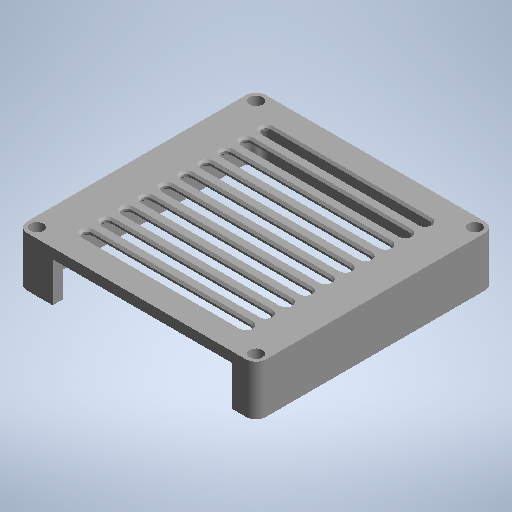
# Autodesk Inventor part: Part6
Saved by Autodesk Inventor 2025.4 (Build 294407000, 407)
## iProperties
Created: 2026-08-04
Part Number: Part6
Material: Générique
Document SubType Name: Modeling
Designer: louis
Density: 1 g/cm^3
Appearance: Par défaut
Author: louis
Autodesk Inventor part; units mm, degrees
ref_plane "YZ Plane" through (0, 0, 0) normal (1, 0, 0) x (0, 1, 0)
ref_plane "XZ Plane" through (0, 0, 0) normal (0, 1, 0) x (-1, 0, 0)
ref_plane "XY Plane" through (0, 0, 0) normal (0, 0, 1) x (1, 0, 0)
sketch "Sketch2" plane through (0, 0, 0) normal (0, 0, 1) x (1, 0, 0)
  line L0 (-55, -60) -> (55, -60)
  line L1 (60, -55) -> (60, 55)
  line L2 (55, 60) -> (-55, 60)
  line L3 (-60, 55) -> (-60, -55)
  line L4 (-60, -60) -> (60, 60) construction
  line L5 (60, -60) -> (-60, 60) construction
  arc A0 (-55, 60) -> (-60, 55) centre (-55, 55) ccw
  arc A1 (60, 55) -> (55, 60) centre (55, 55) ccw
  arc A2 (55, -60) -> (60, -55) centre (55, -55) ccw
  arc A3 (-60, -55) -> (-55, -60) centre (-55, -55) ccw
  line L6 (-55, 55) -> (55, 55)
  line L7 (55, 55) -> (55, -55)
  line L8 (55, -55) -> (-55, -55)
  line L9 (-55, -55) -> (-55, 55)
  circle A4 centre (-55, 55) radius 4
  circle A5 centre (55, 55) radius 4
  circle A6 centre (55, -55) radius 4
  circle A7 centre (-55, -55) radius 4
  point P0 (0, 0)
  point P1 (-55, -51)
  point P2 (-55, 51)
  point P3 (-51, 55)
  point P4 (51, 55)
  point P5 (55, 51)
  point P6 (55, -51)
  point P7 (51, -55)
  point P8 (-51, -55)
  dimension "d0" = 120
  dimension "d1" = 120
  dimension "d2" = 5
  dimension "d3" = 5
  dimension "d4" = 5
  dimension "d5" = 8
  dimension "d6" = 8
  dimension "d7" = 8
  dimension "d8" = 8
  constraints: 20 end point, 8 centre point, 8 point on circle, 8 point on line, 8 tangent, 4 coincident, 4 parallel, 2 equal radius, 2 midpoint, 2 perpendicular, 1 horizontal, 3 other
  measures "d0" distance of L5.end L4.end
  measures "d1" distance of L4.end L5.start
  measures "d2" radius of A0
  measures "d3" radius of A1
  measures "d4" distance between parallel lines of L2 L6
  measures "d5" diameter of A4
  measures "d6" diameter of A5
  measures "d7" diameter of A6
  measures "d8" diameter of A7
extrude "Extrusion1" add sketch "Sketch2" along normal blind 22 contours A3 L3 A0 L2 A1 L1 A2 L0 | L9 A4 L6 | L6 A4 L9 | A5 L7 L6 | L6 L7 A5 | A7 L8 L9 | L9 L8 A7 | A6 L8 L7 | L7 L8 A6
fillet "Fillet1" radius 4 8 edges at (-55, -51, 11) (-51, 55, 11) (-55, 51, 11) (-51, -55, 11) (51, -55, 11) (55, -51, 11) (55, 51, 11) (51, 55, 11)
sketch "Sketch4" plane through (0, 0, 22) normal (0, 0, 1) x (1, 0, 0)
  arc A0 (55, -60) -> (60, -55) centre (55, -55) ccw projected
  line L0 (60, -55) -> (60, 55) projected
  arc A1 (60, 55) -> (55, 60) centre (55, 55) ccw projected
  line L1 (55, 60) -> (-55, 60) projected
  arc A2 (-55, 60) -> (-60, 55) centre (-55, 55) ccw projected
  line L2 (-60, 55) -> (-60, -55) projected
  arc A3 (-60, -55) -> (-55, -60) centre (-55, -55) ccw projected
  line L3 (-55, -60) -> (55, -60) projected
  line L4 (-55, -48.0718) -> (-55, 48.0718) projected
  arc A4 (-53, 51.5359) -> (-55, 48.0718) centre (-51, 48.0718) ccw projected
  arc A5 (-53, 51.5359) -> (-51.5359, 53) centre (-55, 55) ccw projected
  arc A6 (-48.0718, 55) -> (-51.5359, 53) centre (-48.0718, 51) ccw projected
  line L5 (-48.0718, 55) -> (48.0718, 55) projected
  arc A7 (51.5359, 53) -> (48.0718, 55) centre (48.0718, 51) ccw projected
  arc A8 (51.5359, 53) -> (53, 51.5359) centre (55, 55) ccw projected
  arc A9 (55, 48.0718) -> (53, 51.5359) centre (51, 48.0718) ccw projected
  line L6 (55, 48.0718) -> (55, -48.0718) projected
  arc A10 (53, -51.5359) -> (55, -48.0718) centre (51, -48.0718) ccw projected
  arc A11 (53, -51.5359) -> (51.5359, -53) centre (55, -55) ccw projected
  arc A12 (48.0718, -55) -> (51.5359, -53) centre (48.0718, -51) ccw projected
  line L7 (48.0718, -55) -> (-48.0718, -55) projected
  arc A13 (-51.5359, -53) -> (-48.0718, -55) centre (-48.0718, -51) ccw projected
  arc A14 (-51.5359, -53) -> (-53, -51.5359) centre (-55, -55) ccw projected
  arc A15 (-55, -48.0718) -> (-53, -51.5359) centre (-51, -48.0718) ccw projected
  line L8 (-40, 45) -> (40, 45) construction
  line L9 (-40, 42.75) -> (40, 42.75)
  line L10 (40, 47.25) -> (-40, 47.25)
  arc A16 (-40, 47.25) -> (-40, 42.75) centre (-40, 45) ccw
  arc A17 (40, 42.75) -> (40, 47.25) centre (40, 45) ccw
  line L11 (0, 0) -> (0, 45) construction
  line L12 (40, 37.25) -> (-40, 37.25)
  arc A18 (-40, 37.25) -> (-40, 32.75) centre (-40, 35) ccw
  line L13 (-40, 32.75) -> (40, 32.75)
  arc A19 (40, 32.75) -> (40, 37.25) centre (40, 35) ccw
  line L14 (-40, 35) -> (40, 35) construction
  line L15 (40, 27.25) -> (-40, 27.25)
  arc A20 (-40, 27.25) -> (-40, 22.75) centre (-40, 25) ccw
  line L16 (-40, 22.75) -> (40, 22.75)
  arc A21 (40, 22.75) -> (40, 27.25) centre (40, 25) ccw
  line L17 (-40, 25) -> (40, 25) construction
  line L18 (40, 17.25) -> (-40, 17.25)
  arc A22 (-40, 17.25) -> (-40, 12.75) centre (-40, 15) ccw
  line L19 (-40, 12.75) -> (40, 12.75)
  arc A23 (40, 12.75) -> (40, 17.25) centre (40, 15) ccw
  line L20 (-40, 15) -> (40, 15) construction
  line L21 (40, 7.25) -> (-40, 7.25)
  arc A24 (-40, 7.25) -> (-40, 2.75) centre (-40, 5) ccw
  line L22 (-40, 2.75) -> (40, 2.75)
  arc A25 (40, 2.75) -> (40, 7.25) centre (40, 5) ccw
  line L23 (-40, 5) -> (40, 5) construction
  line L24 (40, -2.75) -> (-40, -2.75)
  arc A26 (-40, -2.75) -> (-40, -7.25) centre (-40, -5) ccw
  line L25 (-40, -7.25) -> (40, -7.25)
  arc A27 (40, -7.25) -> (40, -2.75) centre (40, -5) ccw
  line L26 (-40, -5) -> (40, -5) construction
  line L27 (40, -12.75) -> (-40, -12.75)
  arc A28 (-40, -12.75) -> (-40, -17.25) centre (-40, -15) ccw
  line L28 (-40, -17.25) -> (40, -17.25)
  arc A29 (40, -17.25) -> (40, -12.75) centre (40, -15) ccw
  line L29 (-40, -15) -> (40, -15) construction
  line L30 (40, -22.75) -> (-40, -22.75)
  arc A30 (-40, -22.75) -> (-40, -27.25) centre (-40, -25) ccw
  line L31 (-40, -27.25) -> (40, -27.25)
  arc A31 (40, -27.25) -> (40, -22.75) centre (40, -25) ccw
  line L32 (-40, -25) -> (40, -25) construction
  line L33 (40, -32.75) -> (-40, -32.75)
  arc A32 (-40, -32.75) -> (-40, -37.25) centre (-40, -35) ccw
  line L34 (-40, -37.25) -> (40, -37.25)
  arc A33 (40, -37.25) -> (40, -32.75) centre (40, -35) ccw
  line L35 (-40, -35) -> (40, -35) construction
  line L36 (40, -42.75) -> (-40, -42.75)
  arc A34 (-40, -42.75) -> (-40, -47.25) centre (-40, -45) ccw
  line L37 (-40, -47.25) -> (40, -47.25)
  arc A35 (40, -47.25) -> (40, -42.75) centre (40, -45) ccw
  line L38 (-40, -45) -> (40, -45) construction
  dimension "d12" = 4.5
  dimension "d13" = 80
  dimension "d14" = 45
  dimension "d17" = 10
  constraints: 82 end point, 40 point on circle, 20 centre point, 4 coincident, 4 tangent, 2 vertical, 1 horizontal, 1 midpoint, 1 parallel, 99 other
  measures "d12" diameter of A17
  measures "d13" distance of L8.start L8.end
  measures "d14" distance of L11.start L11.end
  measures "d17" distance of L10.start L12.start
extrude "Extrusion2" add sketch "Sketch4" along normal blind 3 contours L3 A3 L2 A2 L1 A1 L0 A0 | L4 A4 A5 A6 L5 A7 A8 A9 L6 A10 A11 A12 L7 A13 A14 A15
chamfer "Chamfer1" distance 1 angle 45 80 edges at (0, 47.25, 25) (42.25, 45, 25) (0, 42.75, 25) (-42.25, 45, 25) (0, 37.25, 25) (42.25, 35, 25) (0, 32.75, 25) (-42.25, 35, 25) (0, 27.25, 25) (42.25, 25, 25) (0, 22.75, 25) (-42.25, 25, 25) (0, 12.75, 25) (-42.25, 15, 25) (0, 17.25, 25) (42.25, 15, 25) (0, 2.75, 25) (-42.25, 5, 25) (0, 7.25, 25) (42.25, 5, 25) (0, -2.75, 25) (42.25, -5, 25) (0, -7.25, 25) (-42.25, -5, 25) (0, -12.75, 25) (42.25, -15, 25) (0, -17.25, 25) (-42.25, -15, 25) (0, -22.75, 25) (42.25, -25, 25) (0, -27.25, 25) (-42.25, -25, 25) (0, -32.75, 25) (42.25, -35, 25) (0, -37.25, 25) (-42.25, -35, 25) (0, -42.75, 25) (42.25, -45, 25) (0, -47.25, 25) (-42.25, -45, 25) (0, 42.75, 22) (-42.25, 45, 22) (0, 47.25, 22) (42.25, 45, 22) (0, 37.25, 22) (42.25, 35, 22) (0, 32.75, 22) (-42.25, 35, 22) (0, 27.25, 22) (42.25, 25, 22) (0, 22.75, 22) (-42.25, 25, 22) (0, 17.25, 22) (42.25, 15, 22) (0, 12.75, 22) (-42.25, 15, 22) (0, 7.25, 22) (42.25, 5, 22) (0, 2.75, 22) (-42.25, 5, 22) (0, -2.75, 22) (42.25, -5, 22) (0, -7.25, 22) (-42.25, -5, 22) (0, -12.75, 22) (42.25, -15, 22) (0, -17.25, 22) (-42.25, -15, 22) (0, -27.25, 22) (-42.25, -25, 22) (0, -22.75, 22) (42.25, -25, 22) (-42.25, -35, 22) (0, -32.75, 22) (42.25, -35, 22) (0, -37.25, 22) (0, -47.25, 22) (-42.25, -45, 22) (0, -42.75, 22) (42.25, -45, 22)
sketch "Sketch6" plane through (0, 0, 25) normal (0, 0, 1) x (1, 0, 0)
  arc A0 (55, -60) -> (60, -55) centre (55, -55) ccw projected
  line L0 (-55, -60) -> (55, -60) projected
  arc A1 (-60, -55) -> (-55, -60) centre (-55, -55) ccw projected
  line L1 (-60, 55) -> (-60, -55) projected
  arc A2 (-55, 60) -> (-60, 55) centre (-55, 55) ccw projected
  line L2 (55, 60) -> (-55, 60) projected
  arc A3 (60, 55) -> (55, 60) centre (55, 55) ccw projected
  line L3 (60, -55) -> (60, 55) projected
  arc A4 (-55, -48.0718) -> (-53, -51.5359) centre (-51, -48.0718) ccw projected
  arc A5 (-51.5359, -53) -> (-53, -51.5359) centre (-55, -55) ccw projected
  arc A6 (-51.5359, -53) -> (-48.0718, -55) centre (-48.0718, -51) ccw projected
  line L4 (48.0718, -55) -> (-48.0718, -55) projected
  arc A7 (48.0718, -55) -> (51.5359, -53) centre (48.0718, -51) ccw projected
  arc A8 (53, -51.5359) -> (51.5359, -53) centre (55, -55) ccw projected
  arc A9 (53, -51.5359) -> (55, -48.0718) centre (51, -48.0718) ccw projected
  line L5 (55, 48.0718) -> (55, -48.0718) projected
  arc A10 (55, 48.0718) -> (53, 51.5359) centre (51, 48.0718) ccw projected
  arc A11 (51.5359, 53) -> (53, 51.5359) centre (55, 55) ccw projected
  arc A12 (51.5359, 53) -> (48.0718, 55) centre (48.0718, 51) ccw projected
  line L6 (-48.0718, 55) -> (48.0718, 55) projected
  arc A13 (-48.0718, 55) -> (-51.5359, 53) centre (-48.0718, 51) ccw projected
  arc A14 (-53, 51.5359) -> (-51.5359, 53) centre (-55, 55) ccw projected
  arc A15 (-53, 51.5359) -> (-55, 48.0718) centre (-51, 48.0718) ccw projected
  line L7 (-55, -48.0718) -> (-55, 48.0718) projected
  point P0 (0, 0)
  constraints: 4 coincident
hole "Hole2" at (55, 55, 25) at (-55, 55, 25) at (-55, -55, 25) at (55, -55, 25) direction (0, 0, -1) diameter 3.6 end through all counterbore diameter 6.5 counterbore depth 10 clearance for "Socket Head Cap Screw" size "M3" standard "Ansi Metric M Profile"
chamfer "Chamfer2" distance 1.4 angle 45 4 edges at (55, 56.8, 15) (55, -53.2, 15) (-55, -53.2, 15) (-55, 56.8, 15)
sketch "Sketch5" plane through (-55, -60, 0) normal (0, -1, 0) x (1, 0, 0)
  line L0 (12.8413, 0) -> (102.8413, 0)
  line L1 (102.8413, 0) -> (102.8413, 20)
  line L2 (102.8413, 20) -> (12.8413, 20)
  line L3 (12.8413, 20) -> (12.8413, 0)
  line L4 (12.8413, 0) -> (102.8413, 20) construction
  line L5 (102.8413, 0) -> (12.8413, 20) construction
  line L6 (0, 0) -> (110, 0) projected
  point P0 (55, 0)
  point P1 (57.8413, 10)
  dimension "d27" = 90
  dimension "d28" = 20
  constraints: 12 end point, 2 midpoint, 2 parallel, 1 collinear, 1 horizontal, 1 perpendicular
  measures "d27" distance of L1.end L2.end
  measures "d28" distance of L2.end L0.start
extrude "Extrusion3" cut sketch "Sketch5" against normal up to surface (5 mm away)
body "Solid1"
